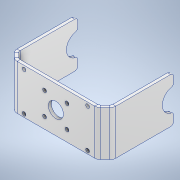
# Autodesk Inventor part: motor_u
Saved by Autodesk Inventor 2020 (Build 240168000, 168)
## iProperties
Created: 2020-08-28
Part Number: motor_u
Material: 알루미늄 6061
Document SubType Name: Sheet Metal
Designer: qwer1
Density: 2.7 g/cm^3
Sheet Metal Rule: 기본값_mm
Appearance: 알루미늄 - 평지
Author: qwer1
Autodesk Inventor part; units mm, degrees
ref_plane "YZ Plane" through (0, 0, 0) normal (1, 0, 0) x (0, 1, 0)
ref_plane "XZ Plane" through (0, 0, 0) normal (0, 1, 0) x (-1, 0, 0)
ref_plane "XY Plane" through (0, 0, 0) normal (0, 0, 1) x (1, 0, 0)
sketch "스케치1" plane through (0, 0, 0) normal (0, 0, 1) x (1, 0, 0)
  circle A0 centre (25.8313, 14.9075) radius 5
  circle A1 centre (18.3313, 22.4075) radius 1.25
  circle A2 centre (18.3313, 7.3526) radius 1.25
  circle A3 centre (33.2769, 22.4075) radius 1.25
  circle A4 centre (46.9521, 27.6627) radius 1.25
  circle A5 centre (46.9521, 2.0974) radius 1.25
  circle A6 centre (33.2769, 7.3526) radius 1.25
  line L0 (25.8041, 29.8443) -> (25.8875, 29.8036)
  line L1 (0, 30) -> (0, 0)
  line L2 (0, 30) -> (51.61, 30)
  line L3 (51.61, 30) -> (51.61, 0)
  line L4 (51.61, 0) -> (0, 0)
  line L5 (0, 0) -> (0, 30)
  circle A7 centre (4.6891, 27.6627) radius 1.25
  circle A8 centre (4.6891, 2.0974) radius 1.25
  dimension "d2" = 10
  dimension "d5" = 2.5
  dimension "d26" = 51.61
  measures "d2" diameter of A0
  measures "d5" diameter of A1
  measures "d26" distance of L3.end L4.end
extrude "판3" add sketch "스케치1" along normal blind 2
sketch "스케치3" plane through (53.0242, 0, -0.5858) normal (0.7071068, 0, 0.7071068) x (0, 1, 0)
  line L0 (30, 0) -> (0, 0)
  line L1 (0, 0) -> (0, -4.3431)
  line L2 (0, -4.3431) -> (30, -4.3431)
  line L3 (30, -4.3431) -> (30, 0)
  constraints: 6 end point, 1 horizontal, 1 perpendicular, 1 vertical
edge flange "플랜지2" height 6 angle 45 thickness 2 bend radius 2 thickness toward (0.7071068, 0, 0.7071068) relief tear relief width 2 relief depth 1 corner gap 2 corner form 0 edges at (51.61, 15, 0) (0, 15, 0) wall of the first edge with corners at (53.0242, 30, -0.5858) (53.0242, 0, -0.5858) (56.0953, 0, -3.6569) (56.0953, 30, -3.6569)
bend "절곡부2"
corner "구석2"
sketch "스케치4" plane through (56.6811, 0, -5.0711) normal (1, 0, 0) x (0, 1, 0)
  line L0 (30, 0) -> (0, 0)
  line L1 (0, 0) -> (0, -38.3431)
  line L2 (0, -38.3431) -> (30, -38.3431)
  line L3 (30, -38.3431) -> (30, 0)
  constraints: 6 end point, 1 horizontal, 1 perpendicular, 1 vertical
edge flange "플랜지3" height 40 angle 45 thickness 2 bend radius 2 thickness toward (1, 0, 0) relief tear relief width 2 relief depth 1 corner gap 2 corner form 0 edges at (56.0953, 15, -3.6569) (-4.4853, 15, -3.6569) wall of the first edge with corners at (56.6811, 30, -5.0711) (56.6811, 0, -5.0711) (56.6811, 0, -43.4142) (56.6811, 30, -43.4142)
bend "절곡부3"
corner "구석3"
sketch "스케치5" plane through (-7.0711, 0, -43.4142) normal (-1, 0, 0) x (0, 0, 1)
  line L0 (0, 30) -> (0, 0) projected
  circle A0 centre (0, 15) radius 7.5
  circle A1 centre (0, 15) radius 14.969
  line L1 (0, 15) -> (14.969, 15)
  point P0 (43.4142, 0)
  point P1 (0, 7.5)
  point P2 (0, 22.5)
  dimension "d48" = 15
  constraints: 2 end point, 1 centre point, 1 coincident, 1 horizontal, 1 horizontal alignment, 1 midpoint, 2 other
  measures "d48" diameter of A0
extrude "돌출2" cut sketch "스케치5" against normal blind 66 contours A0 L1 L0 | L1 A0 L0
fillet "모깎기1" radius 2 8 edges at (57.6811, 0, -43.4142) (-6.0711, 0, -43.4142) (-6.0711, 7.5, -43.4142) (-6.0711, 22.5, -43.4142) (-6.0711, 30, -43.4142) (57.6811, 7.5, -43.4142) (57.6811, 22.5, -43.4142) (57.6811, 30, -43.4142)
equation "\"d28\" = BendReliefWidth"
equation "\"d29\" = BendReliefDepth"
equation "\"d30\" = MinimumRemnant"
equation "\"d31\" = TransitionRadius"
equation "\"d34\" = BendRadius"
equation "\"d35\" = CornerReliefSize"
equation "\"d38\" = BendReliefWidth"
equation "\"d39\" = BendReliefDepth"
equation "\"d40\" = MinimumRemnant"
equation "\"d41\" = TransitionRadius"
equation "\"d44\" = BendRadius"
equation "\"d45\" = CornerReliefSize"
equation "\"TransitionRadius\" = BendRadius"
equation "\"BendReliefWidth\" = 2"
equation "\"BendReliefDepth\" = 1"
equation "\"MinimumRemnant\" = 4"
equation "\"BendRadius\" = 2"
equation "\"CornerReliefSize\" = 8"
